Autodesk Fusion 360 part; units mm, degrees
note: some values were not read from the file. Set by a fixed rule: which sketch regions a step uses.
(part 50 of 59)
  spline S20 degree 5 poles (-24.0278, -3.8184) (-24.0279, -3.8185) (-24.0281, -3.8186) (-24.0283, -3.8188) (-24.0287, -3.8191) (-24.0294, -3.8195) (-24.0301, -3.82) (-24.0309, -3.8206) (-24.0317, -3.8212) (-24.0327, -3.8219) (-24.0338, -3.8227) (-24.035, -3.8235) (-24.0362, -3.8244) (-24.0375, -3.8253) (-24.0389, -3.8263) (-24.0404, -3.8274) (-24.042, -3.8286) (-24.0436, -3.8298) (-24.0453, -3.831) (-24.0471, -3.8324) (-24.049, -3.8338) (-24.051, -3.8352) (-24.053, -3.8367) (-24.0551, -3.8383) (-24.0572, -3.8399) (-24.0595, -3.8416) (-24.0618, -3.8434) (-24.0641, -3.8452) (-24.0666, -3.8471) (-24.0691, -3.849) (-24.0717, -3.851) (-24.0743, -3.853) (-24.077, -3.8551) (-24.0798, -3.8573) (-24.0826, -3.8595) (-24.0855, -3.8618) (-24.0884, -3.8641) (-24.0914, -3.8665) (-24.0945, -3.8689) (-24.0976, -3.8714) (-24.1008, -3.874) (-24.104, -3.8766) (-24.1073, -3.8792) (-24.1107, -3.8819) (-24.1141, -3.8847) (-24.1176, -3.8875) (-24.1211, -3.8904) (-24.1246, -3.8933) (-24.1283, -3.8963) (-24.1319, -3.8994) (-24.1356, -3.9024) (-24.1394, -3.9056) (-24.1432, -3.9088) (-24.1471, -3.912) (-24.151, -3.9153) (-24.155, -3.9187) (-24.159, -3.9221) (-24.1631, -3.9256) (-24.1672, -3.9291) (-24.1713, -3.9326) (-24.1755, -3.9362) (-24.1798, -3.9399) (-24.1841, -3.9436) (-24.1884, -3.9474) (-24.1928, -3.9512) (-24.1972, -3.955) (-24.2017, -3.959) (-24.2062, -3.9629) (-24.2107, -3.9669) (-24.2153, -3.971) (-24.2199, -3.9751) (-24.2246, -3.9793) (-24.2293, -3.9835) (-24.234, -3.9877) (-24.2388, -3.992) (-24.2436, -3.9964) (-24.2485, -4.0008) (-24.2534, -4.0053) (-24.2583, -4.0098) (-24.2633, -4.0143) (-24.2683, -4.0189) (-24.2733, -4.0236) (-24.2784, -4.0282) (-24.2835, -4.033) (-24.2887, -4.0378) (-24.2939, -4.0426) (-24.2991, -4.0475) (-24.3043, -4.0524) (-24.3096, -4.0574) (-24.3149, -4.0624) (-24.3203, -4.0675) (-24.3257, -4.0726) (-24.3311, -4.0778) (-24.3365, -4.083) (-24.342, -4.0882) (-24.3475, -4.0935) (-24.353, -4.0989) (-24.3586, -4.1043) (-24.3642, -4.1097) (-24.3698, -4.1152) (-24.3755, -4.1207) (-24.3812, -4.1263) (-24.3869, -4.1319) (-24.3926, -4.1376) (-24.3984, -4.1433) (-24.4042, -4.1491) (-24.41, -4.1549) (-24.4159, -4.1607) (-24.4218, -4.1666) (-24.4277, -4.1725) (-24.4336, -4.1785) (-24.4395, -4.1845) (-24.4455, -4.1906) (-24.4515, -4.1967) (-24.4576, -4.2029) (-24.4636, -4.2091) (-24.4697, -4.2153) (-24.4758, -4.2216) (-24.482, -4.2279) (-24.4881, -4.2343) (-24.4943, -4.2407) (-24.5005, -4.2472) (-24.5067, -4.2537) (-24.513, -4.2602) (-24.5192, -4.2668) (-24.5255, -4.2735) (-24.5319, -4.2801) (-24.5382, -4.2869) (-24.5446, -4.2936) (-24.5509, -4.3004) (-24.5573, -4.3073) (-24.5638, -4.3142) (-24.5702, -4.3211) (-24.5767, -4.3281) (-24.5831, -4.3351) (-24.5897, -4.3421) (-24.5962, -4.3492) (-24.6027, -4.3564) (-24.6093, -4.3636) (-24.6159, -4.3708) (-24.6225, -4.3781) (-24.6291, -4.3854) (-24.6357, -4.3927) (-24.6424, -4.4001) (-24.6491, -4.4075) (-24.6558, -4.415) (-24.6625, -4.4225) (-24.6692, -4.4301) (-24.6759, -4.4377) (-24.6827, -4.4453) (-24.6895, -4.453) (-24.6963, -4.4607) (-24.7031, -4.4685) (-24.7099, -4.4763) (-24.7168, -4.4841) (-24.7236, -4.492) (-24.7305, -4.4999) (-24.7374, -4.5079) (-24.7443, -4.5159) (-24.7512, -4.5239) (-24.7582, -4.532) (-24.7651, -4.5401) (-24.7721, -4.5483) (-24.7791, -4.5565) (-24.7861, -4.5647) (-24.7931, -4.573) (-24.8001, -4.5813) (-24.8071, -4.5897) (-24.8142, -4.5981) (-24.8212, -4.6065) (-24.8283, -4.615) (-24.8354, -4.6235) (-24.8425, -4.6321) (-24.8496, -4.6407) (-24.8568, -4.6493) (-24.8639, -4.658) (-24.8711, -4.6667) (-24.8782, -4.6754) (-24.8854, -4.6842) (-24.8926, -4.6931) (-24.8998, -4.7019) (-24.907, -4.7108) (-24.9142, -4.7198) (-24.9215, -4.7288) (-24.9287, -4.7378) (-24.936, -4.7469) (-24.9432, -4.7559) (-24.9505, -4.7651) (-24.9578, -4.7743) (-24.9651, -4.7835) (-24.9724, -4.7927) (-24.9797, -4.802) (-24.9871, -4.8113) (-24.9944, -4.8207) (-25.0017, -4.8301) (-25.0091, -4.8395) (-25.0165, -4.849) (-25.0238, -4.8585) (-25.0312, -4.8681) (-25.0386, -4.8777) (-25.046, -4.8873) (-25.0534, -4.897) (-25.0609, -4.9067) (-25.0683, -4.9164) (-25.0757, -4.9262) (-25.0832, -4.936) (-25.0906, -4.9458) (-25.0981, -4.9557) (-25.1055, -4.9657) (-25.113, -4.9756) (-25.1205, -4.9856) (-25.128, -4.9956) (-25.1355, -5.0057) (-25.143, -5.0158) (-25.1505, -5.026) (-25.158, -5.0361) (-25.1655, -5.0464) (-25.1731, -5.0566) (-25.1806, -5.0669) (-25.1881, -5.0772) (-25.1957, -5.0876) (-25.2032, -5.098) (-25.2108, -5.1084) (-25.2184, -5.1189) (-25.2259, -5.1294) (-25.2335, -5.1399) (-25.2411, -5.1505) (-25.2487, -5.1611) (-25.2563, -5.1718) (-25.2639, -5.1825) (-25.2715, -5.1932) (-25.2791, -5.2039) (-25.2867, -5.2147) (-25.2943, -5.2256) (-25.3019, -5.2364) (-25.3096, -5.2473) (-25.3172, -5.2583) (-25.3248, -5.2692) (-25.3325, -5.2802) (-25.3401, -5.2913) (-25.3477, -5.3023) (-25.3539, -5.3112) (-25.3584, -5.3179) (-25.3615, -5.3224) (-25.363, -5.3246) knots 0 0 0 0 0 0 0.00416667 0.00833333 0.0125 0.01666667 0.02083333 0.025 0.02916667 0.03333333 0.0375 0.04166667 0.04583333 0.05 0.05416667 0.05833333 0.0625 0.06666667 0.07083333 0.075 0.07916667 0.08333333 0.0875 0.09166667 0.09583333 0.1 0.10416667 0.10833333 0.1125 0.11666667 0.12083333 0.125 0.12916667 0.13333333 0.1375 0.14166667 0.14583333 0.15 0.15416667 0.15833333 0.1625 0.16666667 0.17083333 0.175 0.17916667 0.18333333 0.1875 0.19166667 0.19583333 0.2 0.20416667 0.20833333 0.2125 0.21666667 0.22083333 0.225 0.22916667 0.23333333 0.2375 0.24166667 0.24583333 0.25 0.25416667 0.25833333 0.2625 0.26666667 0.27083333 0.275 0.27916667 0.28333333 0.2875 0.29166667 0.29583333 0.3 0.30416667 0.30833333 0.3125 0.31666667 0.32083333 0.325 0.32916667 0.33333333 0.3375 0.34166667 0.34583333 0.35 0.35416667 0.35833333 0.3625 0.36666667 0.37083333 0.375 0.37916667 0.38333333 0.3875 0.39166667 0.39583333 0.4 0.40416667 0.40833333 0.4125 0.41666667 0.42083333 0.425 0.42916667 0.43333333 0.4375 0.44166667 0.44583333 0.45 0.45416667 0.45833333 0.4625 0.46666667 0.47083333 0.475 0.47916667 0.48333333 0.4875 0.49166667 0.49583333 0.5 0.50416667 0.50833333 0.5125 0.51666667 0.52083333 0.525 0.52916667 0.53333333 0.5375 0.54166667 0.54583333 0.55 0.55416667 0.55833333 0.5625 0.56666667 0.57083333 0.575 0.57916667 0.58333333 0.5875 0.59166667 0.59583333 0.6 0.60416667 0.60833333 0.6125 0.61666667 0.62083333 0.625 0.62916667 0.63333333 0.6375 0.64166667 0.64583333 0.65 0.65416667 0.65833333 0.6625 0.66666667 0.67083333 0.675 0.67916667 0.68333333 0.6875 0.69166667 0.69583333 0.7 0.70416667 0.70833333 0.7125 0.71666667 0.72083333 0.725 0.72916667 0.73333333 0.7375 0.74166667 0.74583333 0.75 0.75416667 0.75833333 0.7625 0.76666667 0.77083333 0.775 0.77916667 0.78333333 0.7875 0.79166667 0.79583333 0.8 0.80416667 0.80833333 0.8125 0.81666667 0.82083333 0.825 0.82916667 0.83333333 0.8375 0.84166667 0.84583333 0.85 0.85416667 0.85833333 0.8625 0.86666667 0.87083333 0.875 0.87916667 0.88333333 0.8875 0.89166667 0.89583333 0.9 0.90416667 0.90833333 0.9125 0.91666667 0.92083333 0.925 0.92916667 0.93333333 0.9375 0.94166667 0.94583333 0.95 0.95416667 0.95833333 0.9625 0.96666667 0.97083333 0.975 0.97916667 0.98333333 0.9875 0.99166667 0.99583333 1 1 1 1 1 1
  arc A21 (-25.363, -5.3246) -> (-24.7898, -6.1136) centre (0, 12.5) ccw
  spline S21 degree 5 poles (-24.7898, -6.1136) (-24.7872, -6.1128) (-24.782, -6.1113) (-24.7743, -6.109) (-24.7639, -6.1059) (-24.751, -6.1021) (-24.7382, -6.0982) (-24.7253, -6.0943) (-24.7125, -6.0905) (-24.6998, -6.0866) (-24.6871, -6.0827) (-24.6744, -6.0788) (-24.6617, -6.0749) (-24.6491, -6.071) (-24.6365, -6.0671) (-24.624, -6.0632) (-24.6115, -6.0593) (-24.599, -6.0553) (-24.5866, -6.0514) (-24.5742, -6.0475) (-24.5618, -6.0435) (-24.5495, -6.0395) (-24.5372, -6.0356) (-24.5249, -6.0316) (-24.5127, -6.0277) (-24.5005, -6.0237) (-24.4884, -6.0197) (-24.4762, -6.0157) (-24.4642, -6.0117) (-24.4521, -6.0077) (-24.4401, -6.0037) (-24.4281, -5.9997) (-24.4162, -5.9957) (-24.4043, -5.9917) (-24.3925, -5.9877) (-24.3806, -5.9836) (-24.3689, -5.9796) (-24.3571, -5.9756) (-24.3454, -5.9715) (-24.3337, -5.9675) (-24.3221, -5.9634) (-24.3105, -5.9594) (-24.299, -5.9553) (-24.2874, -5.9513) (-24.276, -5.9472) (-24.2645, -5.9431) (-24.2531, -5.9391) (-24.2417, -5.935) (-24.2304, -5.9309) (-24.2191, -5.9269) (-24.2079, -5.9228) (-24.1967, -5.9187) (-24.1855, -5.9146) (-24.1744, -5.9105) (-24.1633, -5.9064) (-24.1522, -5.9023) (-24.1412, -5.8982) (-24.1302, -5.8941) (-24.1193, -5.89) (-24.1084, -5.8859) (-24.0975, -5.8818) (-24.0867, -5.8777) (-24.0759, -5.8736) (-24.0652, -5.8695) (-24.0545, -5.8654) (-24.0438, -5.8613) (-24.0332, -5.8572) (-24.0226, -5.8531) (-24.0121, -5.849) (-24.0016, -5.8449) (-23.9911, -5.8408) (-23.9807, -5.8366) (-23.9703, -5.8325) (-23.96, -5.8284) (-23.9497, -5.8243) (-23.9395, -5.8202) (-23.9292, -5.8161) (-23.9191, -5.812) (-23.909, -5.8079) (-23.8989, -5.8038) (-23.8888, -5.7996) (-23.8788, -5.7955) (-23.8689, -5.7914) (-23.859, -5.7873) (-23.8491, -5.7832) (-23.8393, -5.7791) (-23.8295, -5.775) (-23.8197, -5.7709) (-23.81, -5.7668) (-23.8004, -5.7627) (-23.7907, -5.7587) (-23.7812, -5.7546) (-23.7716, -5.7505) (-23.7622, -5.7464) (-23.7527, -5.7423) (-23.7433, -5.7383) (-23.734, -5.7342) (-23.7247, -5.7301) (-23.7154, -5.726) (-23.7062, -5.722) (-23.697, -5.7179) (-23.6879, -5.7139) (-23.6788, -5.7098) (-23.6697, -5.7058) (-23.6607, -5.7018) (-23.6518, -5.6977) (-23.6429, -5.6937) (-23.634, -5.6897) (-23.6252, -5.6857) (-23.6165, -5.6816) (-23.6077, -5.6776) (-23.5991, -5.6736) (-23.5904, -5.6696) (-23.5818, -5.6657) (-23.5733, -5.6617) (-23.5648, -5.6577) (-23.5564, -5.6537) (-23.548, -5.6498) (-23.5396, -5.6458) (-23.5313, -5.6419) (-23.5231, -5.6379) (-23.5149, -5.634) (-23.5067, -5.6301) (-23.4986, -5.6262) (-23.4905, -5.6223) (-23.4825, -5.6184) (-23.4746, -5.6145) (-23.4666, -5.6106) (-23.4588, -5.6068) (-23.451, -5.6029) (-23.4432, -5.5991) (-23.4355, -5.5952) (-23.4278, -5.5914) (-23.4202, -5.5876) (-23.4126, -5.5838) (-23.4051, -5.58) (-23.3976, -5.5762) (-23.3902, -5.5724) (-23.3828, -5.5687) (-23.3755, -5.5649) (-23.3683, -5.5612) (-23.361, -5.5575) (-23.3539, -5.5538) (-23.3468, -5.5501) (-23.3397, -5.5464) (-23.3327, -5.5427) (-23.3257, -5.539) (-23.3188, -5.5354) (-23.312, -5.5318) (-23.3052, -5.5282) (-23.2984, -5.5246) (-23.2918, -5.521) (-23.2851, -5.5174) (-23.2785, -5.5139) (-23.272, -5.5103) (-23.2655, -5.5068) (-23.2591, -5.5033) (-23.2527, -5.4998) (-23.2464, -5.4963) (-23.2402, -5.4929) (-23.234, -5.4895) (-23.2278, -5.486) (-23.2217, -5.4826) (-23.2157, -5.4793) (-23.2097, -5.4759) (-23.2038, -5.4726) (-23.1979, -5.4692) (-23.1921, -5.4659) (-23.1864, -5.4627) (-23.1807, -5.4594) (-23.1751, -5.4562) (-23.1695, -5.4529) (-23.164, -5.4497) (-23.1585, -5.4466) (-23.1531, -5.4434) (-23.1478, -5.4403) (-23.1425, -5.4372) (-23.1373, -5.4341) (-23.1321, -5.431) (-23.127, -5.428) (-23.122, -5.425) (-23.117, -5.422) (-23.1121, -5.4191) (-23.1072, -5.4161) (-23.1024, -5.4132) (-23.0977, -5.4103) (-23.093, -5.4075) (-23.0884, -5.4047) (-23.0839, -5.4019) (-23.0794, -5.3991) (-23.075, -5.3964) (-23.0706, -5.3937) (-23.0664, -5.391) (-23.0621, -5.3883) (-23.058, -5.3857) (-23.0539, -5.3831) (-23.0499, -5.3806) (-23.0459, -5.3781) (-23.042, -5.3756) (-23.0382, -5.3731) (-23.0344, -5.3707) (-23.0308, -5.3683) (-23.0271, -5.366) (-23.0236, -5.3637) (-23.0201, -5.3614) (-23.0167, -5.3592) (-23.0134, -5.357) (-23.0101, -5.3548) (-23.0069, -5.3527) (-23.0038, -5.3506) (-23.0007, -5.3485) (-22.9978, -5.3465) (-22.9948, -5.3446) (-22.992, -5.3427) (-22.9893, -5.3408) (-22.9866, -5.3389) (-22.984, -5.3372) (-22.9814, -5.3354) (-22.979, -5.3337) (-22.9766, -5.3321) (-22.9743, -5.3305) (-22.9721, -5.3289) (-22.9699, -5.3274) (-22.9679, -5.326) (-22.9659, -5.3246) (-22.964, -5.3232) (-22.9622, -5.3219) (-22.9604, -5.3207) (-22.9588, -5.3195) (-22.9572, -5.3183) (-22.9557, -5.3172) (-22.9543, -5.3162) (-22.953, -5.3153) (-22.9518, -5.3144) (-22.9506, -5.3135) (-22.9496, -5.3127) (-22.9486, -5.312) (-22.9477, -5.3114) (-22.9469, -5.3108) (-22.9463, -5.3103) (-22.9457, -5.3098) (-22.9453, -5.3095) (-22.945, -5.3093) (-22.9448, -5.3092) (-22.9448, -5.3091) knots -1 -1 -1 -1 -1 -1 -0.99583333 -0.99166667 -0.9875 -0.98333333 -0.97916667 -0.975 -0.97083333 -0.96666667 -0.9625 -0.95833333 -0.95416667 -0.95 -0.94583333 -0.94166667 -0.9375 -0.93333333 -0.92916667 -0.925 -0.92083333 -0.91666667 -0.9125 -0.90833333 -0.90416667 -0.9 -0.89583333 -0.89166667 -0.8875 -0.88333333 -0.87916667 -0.875 -0.87083333 -0.86666667 -0.8625 -0.85833333 -0.85416667 -0.85 -0.84583333 -0.84166667 -0.8375 -0.83333333 -0.82916667 -0.825 -0.82083333 -0.81666667 -0.8125 -0.80833333 -0.80416667 -0.8 -0.79583333 -0.79166667 -0.7875 -0.78333333 -0.77916667 -0.775 -0.77083333 -0.76666667 -0.7625 -0.75833333 -0.75416667 -0.75 -0.74583333 -0.74166667 -0.7375 -0.73333333 -0.72916667 -0.725 -0.72083333 -0.71666667 -0.7125 -0.70833333 -0.70416667 -0.7 -0.69583333 -0.69166667 -0.6875 -0.68333333 -0.67916667 -0.675 -0.67083333 -0.66666667 -0.6625 -0.65833333 -0.65416667 -0.65 -0.64583333 -0.64166667 -0.6375 -0.63333333 -0.62916667 -0.625 -0.62083333 -0.61666667 -0.6125 -0.60833333 -0.60416667 -0.6 -0.59583333 -0.59166667 -0.5875 -0.58333333 -0.57916667 -0.575 -0.57083333 -0.56666667 -0.5625 -0.55833333 -0.55416667 -0.55 -0.54583333 -0.54166667 -0.5375 -0.53333333 -0.52916667 -0.525 -0.52083333 -0.51666667 -0.5125 -0.50833333 -0.50416667 -0.5 -0.49583333 -0.49166667 -0.4875 -0.48333333 -0.47916667 -0.475 -0.47083333 -0.46666667 -0.4625 -0.45833333 -0.45416667 -0.45 -0.44583333 -0.44166667 -0.4375 -0.43333333 -0.42916667 -0.425 -0.42083333 -0.41666667 -0.4125 -0.40833333 -0.40416667 -0.4 -0.39583333 -0.39166667 -0.3875 -0.38333333 -0.37916667 -0.375 -0.37083333 -0.36666667 -0.3625 -0.35833333 -0.35416667 -0.35 -0.34583333 -0.34166667 -0.3375 -0.33333333 -0.32916667 -0.325 -0.32083333 -0.31666667 -0.3125 -0.30833333 -0.30416667 -0.3 -0.29583333 -0.29166667 -0.2875 -0.28333333 -0.27916667 -0.275 -0.27083333 -0.26666667 -0.2625 -0.25833333 -0.25416667 -0.25 -0.24583333 -0.24166667 -0.2375 -0.23333333 -0.22916667 -0.225 -0.22083333 -0.21666667 -0.2125 -0.20833333 -0.20416667 -0.2 -0.19583333 -0.19166667 -0.1875 -0.18333333 -0.17916667 -0.175 -0.17083333 -0.16666667 -0.1625 -0.15833333 -0.15416667 -0.15 -0.14583333 -0.14166667 -0.1375 -0.13333333 -0.12916667 -0.125 -0.12083333 -0.11666667 -0.1125 -0.10833333 -0.10416667 -0.1 -0.09583333 -0.09166667 -0.0875 -0.08333333 -0.07916667 -0.075 -0.07083333 -0.06666667 -0.0625 -0.05833333 -0.05416667 -0.05 -0.04583333 -0.04166667 -0.0375 -0.03333333 -0.02916667 -0.025 -0.02083333 -0.01666667 -0.0125 -0.00833333 -0.00416667 0 0 0 0 0 0
  line L43 (-22.9448, -5.3091) -> (-22.9441, -5.3086)
  line L44 (-22.9441, -5.3086) -> (-22.7115, -5.1281)
  arc A22 (-22.7115, -5.1281) -> (-21.9649, -6.0501) centre (0, 12.5) ccw
  line L45 (-21.9649, -6.0501) -> (-22.1898, -6.2401)
  line L46 (-22.1898, -6.2401) -> (-22.1904, -6.2406)
  spline S22 degree 5 poles (-22.1904, -6.2406) (-22.1905, -6.2407) (-22.1907, -6.2408) (-22.1909, -6.241) (-22.1913, -6.2414) (-22.1919, -6.2419) (-22.1925, -6.2424) (-22.1933, -6.2431) (-22.1941, -6.2438) (-22.195, -6.2446) (-22.196, -6.2455) (-22.197, -6.2464) (-22.1982, -6.2474) (-22.1994, -6.2485) (-22.2007, -6.2497) (-22.202, -6.2509) (-22.2035, -6.2522) (-22.205, -6.2536) (-22.2066, -6.255) (-22.2082, -6.2565) (-22.2099, -6.2581) (-22.2117, -6.2597) (-22.2136, -6.2615) (-22.2155, -6.2632) (-22.2175, -6.2651) (-22.2195, -6.267) (-22.2216, -6.269) (-22.2238, -6.271) (-22.226, -6.2732) (-22.2283, -6.2753) (-22.2307, -6.2776) (-22.2331, -6.2799) (-22.2355, -6.2823) (-22.238, -6.2847) (-22.2406, -6.2872) (-22.2433, -6.2897) (-22.2459, -6.2924) (-22.2487, -6.2951) (-22.2515, -6.2978) (-22.2543, -6.3006) (-22.2572, -6.3035) (-22.2602, -6.3064) (-22.2632, -6.3094) (-22.2662, -6.3124) (-22.2693, -6.3156) (-22.2725, -6.3187) (-22.2757, -6.322) (-22.2789, -6.3252) (-22.2822, -6.3286) (-22.2855, -6.332) (-22.2889, -6.3355) (-22.2923, -6.339) (-22.2958, -6.3426) (-22.2993, -6.3462) (-22.3029, -6.3499) (-22.3065, -6.3536) (-22.3101, -6.3574) (-22.3138, -6.3613) (-22.3175, -6.3652) (-22.3212, -6.3692) (-22.325, -6.3732) (-22.3289, -6.3773) (-22.3328, -6.3814) (-22.3367, -6.3856) (-22.3406, -6.3899) (-22.3446, -6.3942) (-22.3486, -6.3986) (-22.3527, -6.403) (-22.3568, -6.4074) (-22.3609, -6.4119) (-22.3651, -6.4165) (-22.3693, -6.4211) (-22.3736, -6.4258) (-22.3778, -6.4306) (-22.3821, -6.4353) (-22.3865, -6.4402) (-22.3909, -6.4451) (-22.3953, -6.45) (-22.3997, -6.455) (-22.4042, -6.46) (-22.4087, -6.4651) (-22.4132, -6.4703) (-22.4177, -6.4755) (-22.4223, -6.4807) (-22.427, -6.486) (-22.4316, -6.4914) (-22.4363, -6.4968) (-22.441, -6.5022) (-22.4457, -6.5077) (-22.4505, -6.5133) (-22.4553, -6.5189) (-22.4601, -6.5246) (-22.4649, -6.5303) (-22.4698, -6.536) (-22.4747, -6.5418) (-22.4796, -6.5477) (-22.4846, -6.5536) (-22.4895, -6.5595) (-22.4945, -6.5655) (-22.4996, -6.5715) (-22.5046, -6.5776) (-22.5097, -6.5838) (-22.5148, -6.59) (-22.5199, -6.5962) (-22.525, -6.6025) (-22.5302, -6.6088) (-22.5354, -6.6152) (-22.5406, -6.6216) (-22.5458, -6.6281) (-22.5511, -6.6346) (-22.5564, -6.6412) (-22.5617, -6.6478) (-22.567, -6.6544) (-22.5723, -6.6611) (-22.5777, -6.6679) (-22.583, -6.6747) (-22.5884, -6.6815) (-22.5939, -6.6884) (-22.5993, -6.6954) (-22.6048, -6.7024) (-22.6102, -6.7094) (-22.6157, -6.7165) (-22.6212, -6.7236) (-22.6268, -6.7307) (-22.6323, -6.7379) (-22.6379, -6.7452) (-22.6435, -6.7525) (-22.6491, -6.7598) (-22.6547, -6.7672) (-22.6603, -6.7747) (-22.666, -6.7821) (-22.6716, -6.7897) (-22.6773, -6.7972) (-22.683, -6.8048) (-22.6887, -6.8125) (-22.6945, -6.8202) (-22.7002, -6.8279) (-22.706, -6.8357) (-22.7118, -6.8436) (-22.7175, -6.8514) (-22.7233, -6.8593) (-22.7292, -6.8673) (-22.735, -6.8753) (-22.7408, -6.8834) (-22.7467, -6.8914) (-22.7526, -6.8996) (-22.7585, -6.9078) (-22.7644, -6.916) (-22.7703, -6.9242) (-22.7762, -6.9325) (-22.7822, -6.9409) (-22.7881, -6.9493) (-22.7941, -6.9577) (-22.8, -6.9662) (-22.806, -6.9747) (-22.812, -6.9832) (-22.818, -6.9918) (-22.8241, -7.0005) (-22.8301, -7.0091) (-22.8361, -7.0179) (-22.8422, -7.0266) (-22.8483, -7.0354) (-22.8543, -7.0443) (-22.8604, -7.0532) (-22.8665, -7.0621) (-22.8726, -7.0711) (-22.8787, -7.0801) (-22.8849, -7.0891) (-22.891, -7.0982) (-22.8971, -7.1073) (-22.9033, -7.1165) (-22.9095, -7.1257) (-22.9156, -7.135) (-22.9218, -7.1443) (-22.928, -7.1536) (-22.9342, -7.163) (-22.9404, -7.1724) (-22.9466, -7.1818) (-22.9528, -7.1913) (-22.9591, -7.2009) (-22.9653, -7.2104) (-22.9715, -7.22) (-22.9778, -7.2297) (-22.984, -7.2394) (-22.9903, -7.2491) (-22.9966, -7.2589) (-23.0029, -7.2687) (-23.0091, -7.2785) (-23.0154, -7.2884) (-23.0217, -7.2984) (-23.028, -7.3083) (-23.0343, -7.3183) (-23.0406, -7.3284) (-23.047, -7.3384) (-23.0533, -7.3486) (-23.0596, -7.3587) (-23.066, -7.3689) (-23.0723, -7.3791) (-23.0786, -7.3894) (-23.085, -7.3997) (-23.0914, -7.4101) (-23.0977, -7.4205) (-23.1041, -7.4309) (-23.1104, -7.4413) (-23.1168, -7.4518) (-23.1232, -7.4624) (-23.1296, -7.473) (-23.136, -7.4836) (-23.1423, -7.4942) (-23.1487, -7.5049) (-23.1551, -7.5156) (-23.1615, -7.5264) (-23.1679, -7.5372) (-23.1743, -7.548) (-23.1807, -7.5589) (-23.1872, -7.5698) (-23.1936, -7.5808) (-23.2, -7.5917) (-23.2064, -7.6028) (-23.2128, -7.6138) (-23.2193, -7.6249) (-23.2257, -7.636) (-23.2321, -7.6472) (-23.2385, -7.6584) (-23.245, -7.6697) (-23.2514, -7.6809) (-23.2578, -7.6922) (-23.2643, -7.7036) (-23.2707, -7.715) (-23.2771, -7.7264) (-23.2836, -7.7379) (-23.29, -7.7493) (-23.2965, -7.7609) (-23.3029, -7.7724) (-23.3094, -7.784) (-23.3158, -7.7957) (-23.3222, -7.8073) (-23.3287, -7.819) (-23.3351, -7.8308) (-23.3416, -7.8426) (-23.348, -7.8544) (-23.3532, -7.8639) (-23.3571, -7.871) (-23.3596, -7.8757) (-23.3609, -7.8781) knots 0 0 0 0 0 0 0.00416667 0.00833333 0.0125 0.01666667 0.02083333 0.025 0.02916667 0.03333333 0.0375 0.04166667 0.04583333 0.05 0.05416667 0.05833333 0.0625 0.06666667 0.07083333 0.075 0.07916667 0.08333333 0.0875 0.09166667 0.09583333 0.1 0.10416667 0.10833333 0.1125 0.11666667 0.12083333 0.125 0.12916667 0.13333333 0.1375 0.14166667 0.14583333 0.15 0.15416667 0.15833333 0.1625 0.16666667 0.17083333 0.175 0.17916667 0.18333333 0.1875 0.19166667 0.19583333 0.2 0.20416667 0.20833333 0.2125 0.21666667 0.22083333 0.225 0.22916667 0.23333333 0.2375 0.24166667 0.24583333 0.25 0.25416667 0.25833333 0.2625 0.26666667 0.27083333 0.275 0.27916667 0.28333333 0.2875 0.29166667 0.29583333 0.3 0.30416667 0.30833333 0.3125 0.31666667 0.32083333 0.325 0.32916667 0.33333333 0.3375 0.34166667 0.34583333 0.35 0.35416667 0.35833333 0.3625 0.36666667 0.37083333 0.375 0.37916667 0.38333333 0.3875 0.39166667 0.39583333 0.4 0.40416667 0.40833333 0.4125 0.41666667 0.42083333 0.425 0.42916667 0.43333333 0.4375 0.44166667 0.44583333 0.45 0.45416667 0.45833333 0.4625 0.46666667 0.47083333 0.475 0.47916667 0.48333333 0.4875 0.49166667 0.49583333 0.5 0.50416667 0.50833333 0.5125 0.51666667 0.52083333 0.525 0.52916667 0.53333333 0.5375 0.54166667 0.54583333 0.55 0.55416667 0.55833333 0.5625 0.56666667 0.57083333 0.575 0.57916667 0.58333333 0.5875 0.59166667 0.59583333 0.6 0.60416667 0.60833333 0.6125 0.61666667 0.62083333 0.625 0.62916667 0.63333333 0.6375 0.64166667 0.64583333 0.65 0.65416667 0.65833333 0.6625 0.66666667 0.67083333 0.675 0.67916667 0.68333333 0.6875 0.69166667 0.69583333 0.7 0.70416667 0.70833333 0.7125 0.71666667 0.72083333 0.725 0.72916667 0.73333333 0.7375 0.74166667 0.74583333 0.75 0.75416667 0.75833333 0.7625 0.76666667 0.77083333 0.775 0.77916667 0.78333333 0.7875 0.79166667 0.79583333 0.8 0.80416667 0.80833333 0.8125 0.81666667 0.82083333 0.825 0.82916667 0.83333333 0.8375 0.84166667 0.84583333 0.85 0.85416667 0.85833333 0.8625 0.86666667 0.87083333 0.875 0.87916667 0.88333333 0.8875 0.89166667 0.89583333 0.9 0.90416667 0.90833333 0.9125 0.91666667 0.92083333 0.925 0.92916667 0.93333333 0.9375 0.94166667 0.94583333 0.95 0.95416667 0.95833333 0.9625 0.96666667 0.97083333 0.975 0.97916667 0.98333333 0.9875 0.99166667 0.99583333 1 1 1 1 1 1
  arc A23 (-23.3609, -7.8781) -> (-22.7084, -8.6029) centre (0, 12.5) ccw
  spline S23 degree 5 poles (-22.7084, -8.6029) (-22.7059, -8.6018) (-22.7009, -8.5998) (-22.6934, -8.5967) (-22.6834, -8.5925) (-22.671, -8.5873) (-22.6586, -8.5822) (-22.6462, -8.577) (-22.6339, -8.5718) (-22.6217, -8.5666) (-22.6094, -8.5614) (-22.5972, -8.5562) (-22.585, -8.551) (-22.5729, -8.5458) (-22.5608, -8.5406) (-22.5487, -8.5354) (-22.5367, -8.5302) (-22.5247, -8.525) (-22.5127, -8.5198) (-22.5008, -8.5145) (-22.4889, -8.5093) (-22.4771, -8.5041) (-22.4653, -8.4989) (-22.4535, -8.4937) (-22.4417, -8.4884) (-22.43, -8.4832) (-22.4184, -8.478) (-22.4067, -8.4727) (-22.3951, -8.4675) (-22.3836, -8.4623) (-22.3721, -8.457) (-22.3606, -8.4518) (-22.3491, -8.4466) (-22.3377, -8.4413) (-22.3264, -8.4361) (-22.315, -8.4308) (-22.3037, -8.4256) (-22.2925, -8.4204) (-22.2812, -8.4151) (-22.2701, -8.4099) (-22.2589, -8.4046) (-22.2478, -8.3994) (-22.2367, -8.3942) (-22.2257, -8.3889) (-22.2147, -8.3837) (-22.2038, -8.3784) (-22.1928, -8.3732) (-22.182, -8.368) (-22.1711, -8.3627) (-22.1603, -8.3575) (-22.1496, -8.3523) (-22.1388, -8.347) (-22.1281, -8.3418) (-22.1175, -8.3366) (-22.1069, -8.3313) (-22.0963, -8.3261) (-22.0858, -8.3209) (-22.0753, -8.3157) (-22.0649, -8.3105) (-22.0544, -8.3052) (-22.0441, -8.3) (-22.0337, -8.2948) (-22.0235, -8.2896) (-22.0132, -8.2844) (-22.003, -8.2792) (-21.9928, -8.274) (-21.9827, -8.2688) (-21.9726, -8.2636) (-21.9625, -8.2584) (-21.9525, -8.2532) (-21.9426, -8.248) (-21.9326, -8.2429) (-21.9228, -8.2377) (-21.9129, -8.2325) (-21.9031, -8.2274) (-21.8933, -8.2222) (-21.8836, -8.217) (-21.8739, -8.2119) (-21.8643, -8.2067) (-21.8547, -8.2016) (-21.8451, -8.1965) (-21.8356, -8.1913) (-21.8261, -8.1862) (-21.8167, -8.1811) (-21.8073, -8.176) (-21.798, -8.1709) (-21.7887, -8.1658) (-21.7794, -8.1607) (-21.7702, -8.1556) (-21.761, -8.1505) (-21.7519, -8.1454) (-21.7428, -8.1404) (-21.7337, -8.1353) (-21.7247, -8.1303) (-21.7158, -8.1252) (-21.7068, -8.1202) (-21.698, -8.1152) (-21.6891, -8.1101) (-21.6803, -8.1051) (-21.6716, -8.1001) (-21.6629, -8.0951) (-21.6542, -8.0902) (-21.6456, -8.0852) (-21.6371, -8.0802) (-21.6285, -8.0753) (-21.6201, -8.0703) (-21.6116, -8.0654) (-21.6032, -8.0605) (-21.5949, -8.0555) (-21.5866, -8.0506) (-21.5783, -8.0457) (-21.5701, -8.0409) (-21.5619, -8.036) (-21.5538, -8.0311) (-21.5458, -8.0263) (-21.5377, -8.0214) (-21.5297, -8.0166) (-21.5218, -8.0118) (-21.5139, -8.007) (-21.5061, -8.0022) (-21.4983, -7.9974) (-21.4905, -7.9927) (-21.4828, -7.9879) (-21.4752, -7.9832) (-21.4676, -7.9784) (-21.46, -7.9737) (-21.4525, -7.969) (-21.445, -7.9644) (-21.4376, -7.9597) (-21.4302, -7.955) (-21.4229, -7.9504) (-21.4156, -7.9458) (-21.4084, -7.9412) (-21.4012, -7.9366) (-21.3941, -7.932) (-21.387, -7.9274) (-21.38, -7.9229) (-21.373, -7.9184) (-21.3661, -7.9139) (-21.3592, -7.9094) (-21.3523, -7.9049) (-21.3455, -7.9004) (-21.3388, -7.896) (-21.3321, -7.8916) (-21.3255, -7.8872) (-21.3189, -7.8828) (-21.3124, -7.8784) (-21.3059, -7.8741) (-21.2995, -7.8698) (-21.2931, -7.8655) (-21.2867, -7.8612) (-21.2805, -7.8569) (-21.2742, -7.8527) (-21.2681, -7.8484) (-21.2619, -7.8442) (-21.2559, -7.8401) (-21.2498, -7.8359) (-21.2439, -7.8318) (-21.238, -7.8277) (-21.2321, -7.8236) (-21.2263, -7.8195) (-21.2205, -7.8155) (-21.2148, -7.8115) (-21.2092, -7.8075) (-21.2036, -7.8035) (-21.1981, -7.7996) (-21.1926, -7.7956) (-21.1871, -7.7918) (-21.1818, -7.7879) (-21.1764, -7.7841) (-21.1712, -7.7802) (-21.166, -7.7765) (-21.1608, -7.7727) (-21.1557, -7.769) (-21.1507, -7.7653) (-21.1457, -7.7616) (-21.1408, -7.758) (-21.1359, -7.7544) (-21.1311, -7.7508) (-21.1263, -7.7472) (-21.1216, -7.7437) (-21.117, -7.7402) (-21.1124, -7.7368) (-21.1079, -7.7333) (-21.1034, -7.73) (-21.099, -7.7266) (-21.0947, -7.7233) (-21.0904, -7.72) (-21.0862, -7.7167) (-21.082, -7.7135) (-21.0779, -7.7103) (-21.0739, -7.7072) (-21.0699, -7.7041) (-21.066, -7.701) (-21.0621, -7.698) (-21.0583, -7.695) (-21.0546, -7.692) (-21.0509, -7.6891) (-21.0473, -7.6862) (-21.0437, -7.6834) (-21.0403, -7.6806) (-21.0368, -7.6778) (-21.0335, -7.6751) (-21.0302, -7.6724) (-21.027, -7.6698) (-21.0238, -7.6672) (-21.0207, -7.6647) (-21.0177, -7.6622) (-21.0148, -7.6597) (-21.0119, -7.6573) (-21.009, -7.655) (-21.0063, -7.6527) (-21.0036, -7.6504) (-21.001, -7.6482) (-20.9984, -7.6461) (-20.996, -7.644) (-20.9936, -7.6419) (-20.9912, -7.6399) (-20.989, -7.638) (-20.9868, -7.6361) (-20.9847, -7.6343) (-20.9826, -7.6325) (-20.9806, -7.6308) (-20.9787, -7.6291) (-20.9769, -7.6275) (-20.9752, -7.626) (-20.9735, -7.6245) (-20.9719, -7.623) (-20.9704, -7.6217) (-20.9689, -7.6204) (-20.9675, -7.6192) (-20.9663, -7.618) (-20.9651, -7.6169) (-20.9639, -7.6159) (-20.9629, -7.6149) (-20.9619, -7.614) (-20.961, -7.6132) (-20.9602, -7.6125) (-20.9595, -7.6118) (-20.9589, -7.6112) (-20.9583, -7.6107) (-20.958, -7.6104) (-20.9577, -7.6102) (-20.9576, -7.61) (-20.9575, -7.61) knots -1 -1 -1 -1 -1 -1 -0.99583333 -0.99166667 -0.9875 -0.98333333 -0.97916667 -0.975 -0.97083333 -0.96666667 -0.9625 -0.95833333 -0.95416667 -0.95 -0.94583333 -0.94166667 -0.9375 -0.93333333 -0.92916667 -0.925 -0.92083333 -0.91666667 -0.9125 -0.90833333 -0.90416667 -0.9 -0.89583333 -0.89166667 -0.8875 -0.88333333 -0.87916667 -0.875 -0.87083333 -0.86666667 -0.8625 -0.85833333 -0.85416667 -0.85 -0.84583333 -0.84166667 -0.8375 -0.83333333 -0.82916667 -0.825 -0.82083333 -0.81666667 -0.8125 -0.80833333 -0.80416667 -0.8 -0.79583333 -0.79166667 -0.7875 -0.78333333 -0.77916667 -0.775 -0.77083333 -0.76666667 -0.7625 -0.75833333 -0.75416667 -0.75 -0.74583333 -0.74166667 -0.7375 -0.73333333 -0.72916667 -0.725 -0.72083333 -0.71666667 -0.7125 -0.70833333 -0.70416667 -0.7 -0.69583333 -0.69166667 -0.6875 -0.68333333 -0.67916667 -0.675 -0.67083333 -0.66666667 -0.6625 -0.65833333 -0.65416667 -0.65 -0.64583333 -0.64166667 -0.6375 -0.63333333 -0.62916667 -0.625 -0.62083333 -0.61666667 -0.6125 -0.60833333 -0.60416667 -0.6 -0.59583333 -0.59166667 -0.5875 -0.58333333 -0.57916667 -0.575 -0.57083333 -0.56666667 -0.5625 -0.55833333 -0.55416667 -0.55 -0.54583333 -0.54166667 -0.5375 -0.53333333 -0.52916667 -0.525 -0.52083333 -0.51666667 -0.5125 -0.50833333 -0.50416667 -0.5 -0.49583333 -0.49166667 -0.4875 -0.48333333 -0.47916667 -0.475 -0.47083333 -0.46666667 -0.4625 -0.45833333 -0.45416667 -0.45 -0.44583333 -0.44166667 -0.4375 -0.43333333 -0.42916667 -0.425 -0.42083333 -0.41666667 -0.4125 -0.40833333 -0.40416667 -0.4 -0.39583333 -0.39166667 -0.3875 -0.38333333 -0.37916667 -0.375 -0.37083333 -0.36666667 -0.3625 -0.35833333 -0.35416667 -0.35 -0.34583333 -0.34166667 -0.3375 -0.33333333 -0.32916667 -0.325 -0.32083333 -0.31666667 -0.3125 -0.30833333 -0.30416667 -0.3 -0.29583333 -0.29166667 -0.2875 -0.28333333 -0.27916667 -0.275 -0.27083333 -0.26666667 -0.2625 -0.25833333 -0.25416667 -0.25 -0.24583333 -0.24166667 -0.2375 -0.23333333 -0.22916667 -0.225 -0.22083333 -0.21666667 -0.2125 -0.20833333 -0.20416667 -0.2 -0.19583333 -0.19166667 -0.1875 -0.18333333 -0.17916667 -0.175 -0.17083333 -0.16666667 -0.1625 -0.15833333 -0.15416667 -0.15 -0.14583333 -0.14166667 -0.1375 -0.13333333 -0.12916667 -0.125 -0.12083333 -0.11666667 -0.1125 -0.10833333 -0.10416667 -0.1 -0.09583333 -0.09166667 -0.0875 -0.08333333 -0.07916667 -0.075 -0.07083333 -0.06666667 -0.0625 -0.05833333 -0.05416667 -0.05 -0.04583333 -0.04166667 -0.0375 -0.03333333 -0.02916667 -0.025 -0.02083333 -0.01666667 -0.0125 -0.00833333 -0.00416667 0 0 0 0 0 0
  line L47 (-20.9575, -7.61) -> (-20.9569, -7.6094)
  line L48 (-20.9569, -7.6094) -> (-20.7445, -7.4055)
  arc A24 (-20.7445, -7.4055) -> (-19.9055, -8.2445) centre (0, 12.5) ccw
  line L49 (-19.9055, -8.2445) -> (-20.1094, -8.4569)
  line L50 (-20.1094, -8.4569) -> (-20.11, -8.4575)
  spline S24 degree 5 poles (-20.11, -8.4575) (-20.11, -8.4576) (-20.1102, -8.4577) (-20.1104, -8.458) (-20.1107, -8.4583) (-20.1112, -8.4589) (-20.1118, -8.4595) (-20.1125, -8.4602) (-20.1132, -8.461) (-20.114, -8.4619) (-20.1149, -8.4629) (-20.1159, -8.4639) (-20.1169, -8.4651) (-20.118, -8.4663) (-20.1192, -8.4675) (-20.1204, -8.4689) (-20.1217, -8.4704) (-20.123, -8.4719) (-20.1245, -8.4735) (-20.126, -8.4752) (-20.1275, -8.4769) (-20.1291, -8.4787) (-20.1308, -8.4806) (-20.1325, -8.4826) (-20.1343, -8.4847) (-20.1361, -8.4868) (-20.138, -8.489) (-20.1399, -8.4912) (-20.1419, -8.4936) (-20.144, -8.496) (-20.1461, -8.4984) (-20.1482, -8.501) (-20.1504, -8.5036) (-20.1527, -8.5063) (-20.155, -8.509) (-20.1573, -8.5119) (-20.1597, -8.5148) (-20.1622, -8.5177) (-20.1647, -8.5207) (-20.1672, -8.5238) (-20.1698, -8.527) (-20.1724, -8.5302) (-20.1751, -8.5335) (-20.1778, -8.5368) (-20.1806, -8.5403) (-20.1834, -8.5437) (-20.1862, -8.5473) (-20.1891, -8.5509) (-20.192, -8.5546) (-20.195, -8.5583) (-20.198, -8.5621) (-20.201, -8.566) (-20.2041, -8.5699) (-20.2072, -8.5739) (-20.2103, -8.5779) (-20.2135, -8.582) (-20.2167, -8.5862) (-20.22, -8.5904) (-20.2233, -8.5947) (-20.2266, -8.599) (-20.23, -8.6034) (-20.2333, -8.6079) (-20.2368, -8.6124) (-20.2402, -8.617) (-20.2437, -8.6216) (-20.2472, -8.6263) (-20.2508, -8.6311) (-20.2544, -8.6359) (-20.258, -8.6408) (-20.2616, -8.6457) (-20.2653, -8.6507) (-20.269, -8.6557) (-20.2727, -8.6608) (-20.2765, -8.666) (-20.2802, -8.6712) (-20.2841, -8.6764) (-20.2879, -8.6818) (-20.2918, -8.6871) (-20.2956, -8.6926) (-20.2996, -8.6981) (-20.3035, -8.7036) (-20.3075, -8.7092) (-20.3115, -8.7148) (-20.3155, -8.7205) (-20.3195, -8.7263) (-20.3236, -8.7321) (-20.3277, -8.738) (-20.3318, -8.7439) (-20.3359, -8.7498) (-20.3401, -8.7559) (-20.3442, -8.7619) (-20.3484, -8.7681) (-20.3527, -8.7742) (-20.3569, -8.7805) (-20.3612, -8.7867) (-20.3655, -8.7931) (-20.3698, -8.7995) (-20.3741, -8.8059) (-20.3784, -8.8124) (-20.3828, -8.8189) (-20.3872, -8.8255) (-20.3916, -8.8321) (-20.396, -8.8388) (-20.4004, -8.8455) (-20.4049, -8.8523) (-20.4094, -8.8592) (-20.4139, -8.8661) (-20.4184, -8.873) (-20.4229, -8.88) (-20.4274, -8.887) (-20.432, -8.8941) (-20.4366, -8.9012) (-20.4412, -8.9084) (-20.4458, -8.9156) (-20.4504, -8.9229) (-20.455, -8.9302) (-20.4597, -8.9376) (-20.4644, -8.945) (-20.469, -8.9525) (-20.4737, -8.96) (-20.4784, -8.9676) (-20.4832, -8.9752) (-20.4879, -8.9828) (-20.4927, -8.9905) (-20.4974, -8.9983) (-20.5022, -9.0061) (-20.507, -9.0139) (-20.5118, -9.0218) (-20.5166, -9.0297) (-20.5214, -9.0377) (-20.5263, -9.0458) (-20.5311, -9.0538) (-20.536, -9.0619) (-20.5409, -9.0701) (-20.5457, -9.0783) (-20.5506, -9.0866) (-20.5555, -9.0949) (-20.5605, -9.1032) (-20.5654, -9.1116) (-20.5703, -9.1201) (-20.5753, -9.1285) (-20.5802, -9.1371) (-20.5852, -9.1456) (-20.5902, -9.1542) (-20.5951, -9.1629) (-20.6001, -9.1716) (-20.6051, -9.1803) (-20.6101, -9.1891) (-20.6152, -9.198) (-20.6202, -9.2068) (-20.6252, -9.2158) (-20.6303, -9.2247) (-20.6353, -9.2337) (-20.6404, -9.2428) (-20.6454, -9.2519) (-20.6505, -9.261) (-20.6556, -9.2702) (-20.6607, -9.2794) (-20.6658, -9.2887) (-20.6709, -9.298) (-20.676, -9.3073) (-20.6811, -9.3167) (-20.6862, -9.3261) (-20.6913, -9.3356) (-20.6965, -9.3451) (-20.7016, -9.3547) (-20.7067, -9.3643) (-20.7119, -9.3739) (-20.717, -9.3836) (-20.7222, -9.3933) (-20.7274, -9.4031) (-20.7325, -9.4129) (-20.7377, -9.4228) (-20.7429, -9.4326) (-20.748, -9.4426) (-20.7532, -9.4525) (-20.7584, -9.4625) (-20.7636, -9.4726) (-20.7688, -9.4827) (-20.774, -9.4928) (-20.7792, -9.503) (-20.7844, -9.5132) (-20.7896, -9.5235) (-20.7948, -9.5337) (-20.8, -9.5441) (-20.8052, -9.5544) (-20.8105, -9.5649) (-20.8157, -9.5753) (-20.8209, -9.5858) (-20.8261, -9.5963) (-20.8313, -9.6069) (-20.8366, -9.6175) (-20.8418, -9.6281) (-20.847, -9.6388) (-20.8523, -9.6496) (-20.8575, -9.6603) (-20.8627, -9.6711) (-20.868, -9.682) (-20.8732, -9.6928) (-20.8784, -9.7038) (-20.8837, -9.7147) (-20.8889, -9.7257) (-20.8942, -9.7367) (-20.8994, -9.7478) (-20.9046, -9.7589) (-20.9099, -9.7701) (-20.9151, -9.7812) (-20.9204, -9.7925) (-20.9256, -9.8037) (-20.9308, -9.815) (-20.9361, -9.8264) (-20.9413, -9.8377) (-20.9466, -9.8491) (-20.9518, -9.8606) (-20.957, -9.8721) (-20.9623, -9.8836) (-20.9675, -9.8951) (-20.9727, -9.9067) (-20.978, -9.9184) (-20.9832, -9.93) (-20.9884, -9.9417) (-20.9937, -9.9535) (-20.9989, -9.9653) (-21.0041, -9.9771) (-21.0093, -9.9889) (-21.0145, -10.0008) (-21.0198, -10.0127) (-21.025, -10.0247) (-21.0302, -10.0367) (-21.0354, -10.0487) (-21.0406, -10.0608) (-21.0458, -10.0729) (-21.051, -10.085) (-21.0562, -10.0972) (-21.0614, -10.1094) (-21.0666, -10.1217) (-21.0718, -10.1339) (-21.077, -10.1462) (-21.0822, -10.1586) (-21.0873, -10.171) (-21.0925, -10.1834) (-21.0967, -10.1934) (-21.0998, -10.2009) (-21.1018, -10.2059) (-21.1029, -10.2084) knots 0 0 0 0 0 0 0.00416667 0.00833333 0.0125 0.01666667 0.02083333 0.025 0.02916667 0.03333333 0.0375 0.04166667 0.04583333 0.05 0.05416667 0.05833333 0.0625 0.06666667 0.07083333 0.075 0.07916667 0.08333333 0.0875 0.09166667 0.09583333 0.1 0.10416667 0.10833333 0.1125 0.11666667 0.12083333 0.125 0.12916667 0.13333333 0.1375 0.14166667 0.14583333 0.15 0.15416667 0.15833333 0.1625 0.16666667 0.17083333 0.175 0.17916667 0.18333333 0.1875 0.19166667 0.19583333 0.2 0.20416667 0.20833333 0.2125 0.21666667 0.22083333 0.225 0.22916667 0.23333333 0.2375 0.24166667 0.24583333 0.25 0.25416667 0.25833333 0.2625 0.26666667 0.27083333 0.275 0.27916667 0.28333333 0.2875 0.29166667 0.29583333 0.3 0.30416667 0.30833333 0.3125 0.31666667 0.32083333 0.325 0.32916667 0.33333333 0.3375 0.34166667 0.34583333 0.35 0.35416667 0.35833333 0.3625 0.36666667 0.37083333 0.375 0.37916667 0.38333333 0.3875 0.39166667 0.39583333 0.4 0.40416667 0.40833333 0.4125 0.41666667 0.42083333 0.425 0.42916667 0.43333333 0.4375 0.44166667 0.44583333 0.45 0.45416667 0.45833333 0.4625 0.46666667 0.47083333 0.475 0.47916667 0.48333333 0.4875 0.49166667 0.49583333 0.5 0.50416667 0.50833333 0.5125 0.51666667 0.52083333 0.525 0.52916667 0.53333333 0.5375 0.54166667 0.54583333 0.55 0.55416667 0.55833333 0.5625 0.56666667 0.57083333 0.575 0.57916667 0.58333333 0.5875 0.59166667 0.59583333 0.6 0.60416667 0.60833333 0.6125 0.61666667 0.62083333 0.625 0.62916667 0.63333333 0.6375 0.64166667 0.64583333 0.65 0.65416667 0.65833333 0.6625 0.66666667 0.67083333 0.675 0.67916667 0.68333333 0.6875 0.69166667 0.69583333 0.7 0.70416667 0.70833333 0.7125 0.71666667 0.72083333 0.725 0.72916667 0.73333333 0.7375 0.74166667 0.74583333 0.75 0.75416667 0.75833333 0.7625 0.76666667 0.77083333 0.775 0.77916667 0.78333333 0.7875 0.79166667 0.79583333 0.8 0.80416667 0.80833333 0.8125 0.81666667 0.82083333 0.825 0.82916667 0.83333333 0.8375 0.84166667 0.84583333 0.85 0.85416667 0.85833333 0.8625 0.86666667 0.87083333 0.875 0.87916667 0.88333333 0.8875 0.89166667 0.89583333 0.9 0.90416667 0.90833333 0.9125 0.91666667 0.92083333 0.925 0.92916667 0.93333333 0.9375 0.94166667 0.94583333 0.95 0.95416667 0.95833333 0.9625 0.96666667 0.97083333 0.975 0.97916667 0.98333333 0.9875 0.99166667 0.99583333 1 1 1 1 1 1
  arc A25 (-21.1029, -10.2084) -> (-20.3781, -10.8609) centre (0, 12.5) ccw
  spline S25 degree 5 poles (-20.3781, -10.8609) (-20.3757, -10.8596) (-20.371, -10.8571) (-20.3639, -10.8532) (-20.3544, -10.848) (-20.3426, -10.8416) (-20.3308, -10.8351) (-20.319, -10.8287) (-20.3073, -10.8222) (-20.2957, -10.8158) (-20.284, -10.8094) (-20.2724, -10.8029) (-20.2609, -10.7965) (-20.2493, -10.79) (-20.2379, -10.7836) (-20.2264, -10.7771) (-20.215, -10.7707) (-20.2036, -10.7643) (-20.1922, -10.7578) (-20.1809, -10.7514) (-20.1697, -10.745) (-20.1584, -10.7385) (-20.1472, -10.7321) (-20.136, -10.7257) (-20.1249, -10.7193) (-20.1138, -10.7128) (-20.1028, -10.7064) (-20.0917, -10.7) (-20.0808, -10.6936) (-20.0698, -10.6872) (-20.0589, -10.6807) (-20.048, -10.6743) (-20.0372, -10.6679) (-20.0264, -10.6615) (-20.0156, -10.6551) (-20.0049, -10.6487) (-19.9942, -10.6423) (-19.9836, -10.636) (-19.973, -10.6296) (-19.9624, -10.6232) (-19.9518, -10.6168) (-19.9413, -10.6104) (-19.9309, -10.6041) (-19.9205, -10.5977) (-19.9101, -10.5914) (-19.8997, -10.585) (-19.8894, -10.5786) (-19.8791, -10.5723) (-19.8689, -10.566) (-19.8587, -10.5596) (-19.8486, -10.5533) (-19.8384, -10.547) (-19.8284, -10.5406) (-19.8183, -10.5343) (-19.8083, -10.528) (-19.7984, -10.5217) (-19.7884, -10.5154) (-19.7785, -10.5091) (-19.7687, -10.5029) (-19.7589, -10.4966) (-19.7491, -10.4903) (-19.7394, -10.484) (-19.7297, -10.4778) (-19.72, -10.4715) (-19.7104, -10.4653) (-19.7009, -10.4591) (-19.6913, -10.4528) (-19.6818, -10.4466) (-19.6724, -10.4404) (-19.663, -10.4342) (-19.6536, -10.428) (-19.6443, -10.4218) (-19.635, -10.4156) (-19.6257, -10.4095) (-19.6165, -10.4033) (-19.6073, -10.3971) (-19.5982, -10.391) (-19.5891, -10.3849) (-19.5801, -10.3787) (-19.5711, -10.3726) (-19.5621, -10.3665) (-19.5532, -10.3604) (-19.5443, -10.3543) (-19.5354, -10.3483) (-19.5266, -10.3422) (-19.5179, -10.3361) (-19.5091, -10.3301) (-19.5005, -10.3241) (-19.4918, -10.318) (-19.4832, -10.312) (-19.4747, -10.306) (-19.4662, -10.3) (-19.4577, -10.2941) (-19.4493, -10.2881) (-19.4409, -10.2822) (-19.4325, -10.2762) (-19.4242, -10.2703) (-19.416, -10.2644) (-19.4078, -10.2585) (-19.3996, -10.2526) (-19.3914, -10.2467) (-19.3834, -10.2408) (-19.3753, -10.235) (-19.3673, -10.2292) (-19.3593, -10.2233) (-19.3514, -10.2175) (-19.3436, -10.2118) (-19.3357, -10.206) (-19.3279, -10.2002) (-19.3202, -10.1945) (-19.3125, -10.1887) (-19.3048, -10.183) (-19.2972, -10.1773) (-19.2897, -10.1716) (-19.2821, -10.166) (-19.2747, -10.1603) (-19.2672, -10.1547) (-19.2598, -10.1491) (-19.2525, -10.1435) (-19.2452, -10.1379) (-19.2379, -10.1323) (-19.2307, -10.1268) (-19.2236, -10.1212) (-19.2165, -10.1157) (-19.2094, -10.1102) (-19.2024, -10.1048) (-19.1954, -10.0993) (-19.1884, -10.0939) (-19.1815, -10.0884) (-19.1747, -10.083) (-19.1679, -10.0777) (-19.1611, -10.0723) (-19.1544, -10.067) (-19.1478, -10.0617) (-19.1412, -10.0564) (-19.1346, -10.0511) (-19.1281, -10.0458) (-19.1216, -10.0406) (-19.1152, -10.0354) (-19.1088, -10.0302) (-19.1025, -10.025) (-19.0962, -10.0199) (-19.09, -10.0148) (-19.0838, -10.0097) (-19.0776, -10.0046) (-19.0715, -9.9996) (-19.0655, -9.9945) (-19.0595, -9.9895) (-19.0536, -9.9846) (-19.0477, -9.9796) (-19.0418, -9.9747) (-19.036, -9.9698) (-19.0303, -9.9649) (-19.0246, -9.9601) (-19.0189, -9.9553) (-19.0133, -9.9505) (-19.0077, -9.9457) (-19.0022, -9.941) (-18.9968, -9.9363) (-18.9914, -9.9316) (-18.986, -9.927) (-18.9807, -9.9223) (-18.9755, -9.9177) (-18.9703, -9.9132) (-18.9651, -9.9087) (-18.96, -9.9042) (-18.955, -9.8997) (-18.95, -9.8953) (-18.9451, -9.8909) (-18.9402, -9.8865) (-18.9353, -9.8821) (-18.9306, -9.8778) (-18.9258, -9.8736) (-18.9211, -9.8693) (-18.9165, -9.8651) (-18.9119, -9.8609) (-18.9074, -9.8568) (-18.903, -9.8527) (-18.8986, -9.8486) (-18.8942, -9.8446) (-18.8899, -9.8406) (-18.8856, -9.8367) (-18.8814, -9.8328) (-18.8773, -9.8289) (-18.8732, -9.825) (-18.8692, -9.8212) (-18.8652, -9.8175) (-18.8613, -9.8138) (-18.8574, -9.8101) (-18.8536, -9.8065) (-18.8499, -9.8029) (-18.8462, -9.7993) (-18.8426, -9.7958) (-18.839, -9.7923) (-18.8355, -9.7889) (-18.832, -9.7855) (-18.8286, -9.7822) (-18.8252, -9.7789) (-18.822, -9.7757) (-18.8187, -9.7725) (-18.8156, -9.7693) (-18.8124, -9.7662) (-18.8094, -9.7632) (-18.8064, -9.7602) (-18.8035, -9.7572) (-18.8006, -9.7543) (-18.7978, -9.7515) (-18.7951, -9.7487) (-18.7924, -9.7459) (-18.7897, -9.7433) (-18.7872, -9.7406) (-18.7847, -9.738) (-18.7823, -9.7355) (-18.7799, -9.7331) (-18.7776, -9.7307) (-18.7753, -9.7283) (-18.7732, -9.726) (-18.771, -9.7238) (-18.769, -9.7216) (-18.767, -9.7195) (-18.7651, -9.7175) (-18.7632, -9.7155) (-18.7615, -9.7136) (-18.7597, -9.7117) (-18.7581, -9.7099) (-18.7565, -9.7082) (-18.755, -9.7066) (-18.7536, -9.705) (-18.7522, -9.7035) (-18.7509, -9.702) (-18.7497, -9.7007) (-18.7485, -9.6994) (-18.7474, -9.6982) (-18.7464, -9.697) (-18.7455, -9.696) (-18.7446, -9.695) (-18.7438, -9.6941) (-18.7431, -9.6933) (-18.7424, -9.6925) (-18.7419, -9.6919) (-18.7414, -9.6913) (-18.741, -9.6909) (-18.7408, -9.6907) (-18.7407, -9.6905) (-18.7406, -9.6904) knots -1 -1 -1 -1 -1 -1 -0.99583333 -0.99166667 -0.9875 -0.98333333 -0.97916667 -0.975 -0.97083333 -0.96666667 -0.9625 -0.95833333 -0.95416667 -0.95 -0.94583333 -0.94166667 -0.9375 -0.93333333 -0.92916667 -0.925 -0.92083333 -0.91666667 -0.9125 -0.90833333 -0.90416667 -0.9 -0.89583333 -0.89166667 -0.8875 -0.88333333 -0.87916667 -0.875 -0.87083333 -0.86666667 -0.8625 -0.85833333 -0.85416667 -0.85 -0.84583333 -0.84166667 -0.8375 -0.83333333 -0.82916667 -0.825 -0.82083333 -0.81666667 -0.8125 -0.80833333 -0.80416667 -0.8 -0.79583333 -0.79166667 -0.7875 -0.78333333 -0.77916667 -0.775 -0.77083333 -0.76666667 -0.7625 -0.75833333 -0.75416667 -0.75 -0.74583333 -0.74166667 -0.7375 -0.73333333 -0.72916667 -0.725 -0.72083333 -0.71666667 -0.7125 -0.70833333 -0.70416667 -0.7 -0.69583333 -0.69166667 -0.6875 -0.68333333 -0.67916667 -0.675 -0.67083333 -0.66666667 -0.6625 -0.65833333 -0.65416667 -0.65 -0.64583333 -0.64166667 -0.6375 -0.63333333 -0.62916667 -0.625 -0.62083333 -0.61666667 -0.6125 -0.60833333 -0.60416667 -0.6 -0.59583333 -0.59166667 -0.5875 -0.58333333 -0.57916667 -0.575 -0.57083333 -0.56666667 -0.5625 -0.55833333 -0.55416667 -0.55 -0.54583333 -0.54166667 -0.5375 -0.53333333 -0.52916667 -0.525 -0.52083333 -0.51666667 -0.5125 -0.50833333 -0.50416667 -0.5 -0.49583333 -0.49166667 -0.4875 -0.48333333 -0.47916667 -0.475 -0.47083333 -0.46666667 -0.4625 -0.45833333 -0.45416667 -0.45 -0.44583333 -0.44166667 -0.4375 -0.43333333 -0.42916667 -0.425 -0.42083333 -0.41666667 -0.4125 -0.40833333 -0.40416667 -0.4 -0.39583333 -0.39166667 -0.3875 -0.38333333 -0.37916667 -0.375 -0.37083333 -0.36666667 -0.3625 -0.35833333 -0.35416667 -0.35 -0.34583333 -0.34166667 -0.3375 -0.33333333 -0.32916667 -0.325 -0.32083333 -0.31666667 -0.3125 -0.30833333 -0.30416667 -0.3 -0.29583333 -0.29166667 -0.2875 -0.28333333 -0.27916667 -0.275 -0.27083333 -0.26666667 -0.2625 -0.25833333 -0.25416667 -0.25 -0.24583333 -0.24166667 -0.2375 -0.23333333 -0.22916667 -0.225 -0.22083333 -0.21666667 -0.2125 -0.20833333 -0.20416667 -0.2 -0.19583333 -0.19166667 -0.1875 -0.18333333 -0.17916667 -0.175 -0.17083333 -0.16666667 -0.1625 -0.15833333 -0.15416667 -0.15 -0.14583333 -0.14166667 -0.1375 -0.13333333 -0.12916667 -0.125 -0.12083333 -0.11666667 -0.1125 -0.10833333 -0.10416667 -0.1 -0.09583333 -0.09166667 -0.0875 -0.08333333 -0.07916667 -0.075 -0.07083333 -0.06666667 -0.0625 -0.05833333 -0.05416667 -0.05 -0.04583333 -0.04166667 -0.0375 -0.03333333 -0.02916667 -0.025 -0.02083333 -0.01666667 -0.0125 -0.00833333 -0.00416667 0 0 0 0 0 0
  line L51 (-18.7406, -9.6904) -> (-18.7401, -9.6898)
  line L52 (-18.7401, -9.6898) -> (-18.5501, -9.4649)
  arc A26 (-18.5501, -9.4649) -> (-17.6281, -10.2115) centre (0, 12.5) ccw
  line L53 (-17.6281, -10.2115) -> (-17.8086, -10.4441)
  line L54 (-17.8086, -10.4441) -> (-17.8091, -10.4448)